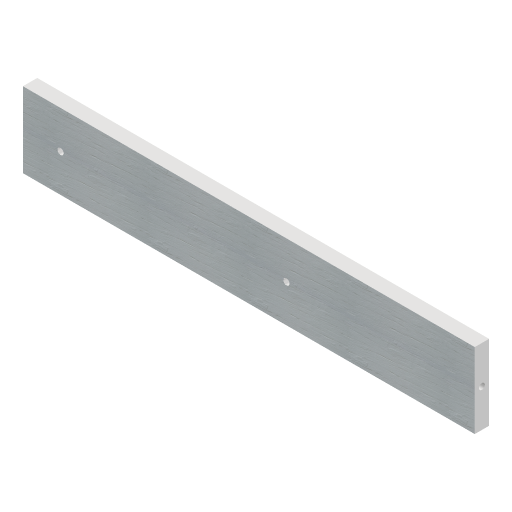
# Autodesk Inventor part: C
Saved by Autodesk Inventor 2024 (Build 280153000, 153)
## iProperties
Created: 2024-03-20
Part Number: C
Material: Generic
Document SubType Name: Modeling
Designer: marco
Density: 1 g/cm^3
Appearance: Default
Author: marco
Autodesk Inventor part; units mm, degrees
ref_plane "YZ Plane" through (0, 0, 0) normal (1, 0, 0) x (0, 1, 0)
ref_plane "XZ Plane" through (0, 0, 0) normal (0, 1, 0) x (-1, 0, 0)
ref_plane "XY Plane" through (0, 0, 0) normal (0, 0, 1) x (1, 0, 0)
sketch "Sketch1" plane through (0, 0, 0) normal (0, 0, 1) x (1, 0, 0)
  line L0 (300, -50) -> (-300, -50)
  line L1 (-300, -50) -> (-300, 50)
  line L2 (-300, 50) -> (300, 50)
  line L3 (300, 50) -> (300, -50)
  line L4 (300, -50) -> (-300, 50) construction
  line L5 (-300, -50) -> (300, 50) construction
  point P0 (0, 0)
  dimension "d0" = 600
  dimension "d1" = 100
  constraints: 12 end point, 2 midpoint, 2 parallel, 1 horizontal, 1 perpendicular
  measures "d0" distance of L1.end L2.end
  measures "d1" distance of L0.end L1.end
extrude "Extrusion1" add sketch "Sketch1" along normal blind 9.5 and the other way blind 9.5
sketch "Sketch2" plane through (0, 0, 9.5) normal (0, 0, 1) x (1, 0, 0)
  line L0 (300, -50) -> (300, 50) projected
  line L1 (300, 0) -> (50, 0)
  line L2 (-300, 50) -> (-300, -50) projected
  line L3 (-300, 0) -> (-250, 0)
  circle A0 centre (-250, 0) radius 4
  circle A1 centre (50, 0) radius 4
  point P0 (0, 0)
  dimension "d6" = 250
  dimension "d7" = 50
  dimension "d8" = 8
  dimension "d9" = 8
  constraints: 4 end point, 2 centre point, 2 coincident, 2 horizontal, 2 midpoint
  measures "d6" distance of L1.start L1.end
  measures "d7" distance of L3.start L3.end
  measures "d8" diameter of A0
  measures "d9" diameter of A1
extrude "Extrusion2" cut sketch "Sketch2" against normal blind 11
sketch "Sketch3" plane through (300, -50, 9.5) normal (1, 0, 0) x (0, 0, -1)
  circle A0 centre (9.5, 50) radius 4
  dimension "d12" = 8
  constraints: 1 centre point, 1 coincident
  measures "d12" diameter of A0
extrude "Extrusion3" cut sketch "Sketch3" against normal blind 11
sketch "Sketch4" plane through (-300, -50, 9.5) normal (-1, 0, 0) x (0, 0, 1)
  circle A0 centre (-9.5, 50) radius 4
  dimension "d15" = 8
  constraints: 1 centre point, 1 coincident
  measures "d15" diameter of A0
extrude "Extrusion4" cut sketch "Sketch4" against normal blind 11
sketch "Sketch5" plane through (-300, -50, 9.5) normal (0, -1, 0) x (1, 0, 0)
  line L0 (0, -19) -> (0, 0) projected
  line L1 (0, -9.5) -> (50, -9.5)
  line L2 (50, -9.5) -> (216.6667, -9.5)
  line L3 (216.6667, -9.5) -> (383.3333, -9.5)
  line L4 (383.3333, -9.5) -> (550, -9.5)
  line L5 (550, -9.5) -> (600, -9.5)
  circle A0 centre (50, -9.5) radius 4
  circle A1 centre (216.6667, -9.5) radius 4
  circle A2 centre (383.3333, -9.5) radius 4
  circle A3 centre (550, -9.5) radius 4
  point P0 (300, -9.5)
  dimension "d18" = 50
  dimension "d19" = 166.6667
  dimension "d20" = 166.6667
  dimension "d21" = 166.6667
  dimension "d22" = 50
  dimension "d23" = 8
  dimension "d24" = 8
  dimension "d25" = 8
  dimension "d26" = 8
  constraints: 10 end point, 4 centre point, 4 coincident, 4 point on line, 1 horizontal, 1 midpoint
  measures "d18" distance of L1.start L1.end
  measures "d19" distance of L1.end L2.end
  measures "d20" distance of L2.end L3.end
  measures "d21" distance of L3.end L4.end
  measures "d22" distance of L4.end L5.end
  measures "d23" diameter of A0
  measures "d24" diameter of A1
  measures "d25" diameter of A2
  measures "d26" diameter of A3
extrude "Extrusion5" cut sketch "Sketch5" against normal blind 11
body "Solid1"
